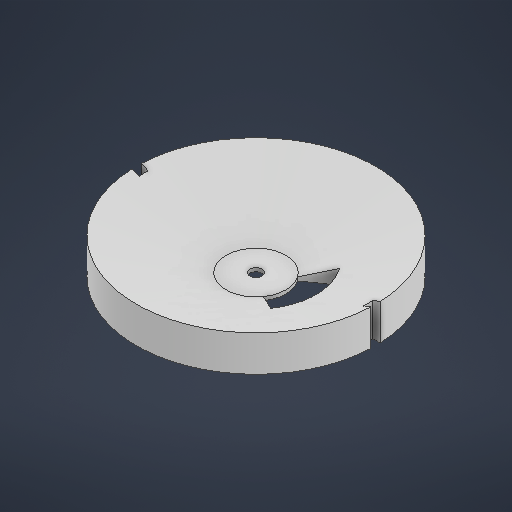
# Autodesk Inventor part: feeder
Saved by Autodesk Inventor 2025.1 (Build 291241020, 241B)
## iProperties
Created: 2024-09-17
Part Number: feeder
Material: Generic
Document SubType Name: Modeling
Designer: maxim
Density: 1 g/cm^3
Appearance: Default
Author: maxim
Autodesk Inventor part; units mm, degrees
ref_plane "YZ Plane" through (0, 0, 0) normal (1, 0, 0) x (0, 1, 0)
ref_plane "XZ Plane" through (0, 0, 0) normal (0, 1, 0) x (-1, 0, 0)
ref_plane "XY Plane" through (0, 0, 0) normal (0, 0, 1) x (1, 0, 0)
sketch "Sketch2" plane through (0, 0, 0) normal (0, 0, 1) x (1, 0, 0)
  line L0 (-50, 0) -> (-99.9, 0)
  line L1 (-99.9, 0) -> (-99.9, 30)
  line L2 (0, 0) -> (0, 50.0549)
  line L3 (-99.9, 30) -> (-25, 3)
  line L4 (-50, 0) -> (0, 0)
  line L5 (-25, 3) -> (0, 3)
  line L6 (0, 3) -> (0, 0)
  point P0 (-99.9, 15)
  dimension "d2" = 30
  dimension "d6" = 199.8
  dimension "d15" = 50
  dimension "d16" = 3
  constraints: 14 end point, 2 horizontal, 2 vertical, 1 collinear, 1 midpoint, 1 perpendicular, 1 point on line
  measures "d2" distance of L0.end L1.end
  measures "d6" diameter of point (-99.9, 15) L2
  measures "d15" diameter of L3.end L2
  measures "d16" distance of L2.start L5.end
revolve "Revolution1" add sketch "Sketch2" angle 360 about axis through (0, 0, 0) along (0, 1, 0)
sketch "Sketch3" plane through (0, 0, 0) normal (0, -1, 0) x (1, 0, 0)
  circle A0 centre (0, 0) radius 99.9 projected
  line L0 (0, 0) -> (99.8199, 4)
  line L1 (0, 0) -> (99.8199, -4)
  line L2 (0, 0) -> (99.9, 0) construction
  line L3 (11.4718, 0) -> (11.4718, -0.4597) construction
  line L4 (11.4718, 0) -> (11.4718, 0.4597) construction
  circle A1 centre (0, 0) radius 93.9
  point P0 (93.8247, 3.7598)
  point P1 (93.8247, -3.7598)
  dimension "d8" = 8
  dimension "d9" = 6
  constraints: 10 end point, 4 point on line, 3 point on circle, 1 centre point, 1 coincident, 1 collinear, 1 horizontal, 1 vertical
  measures "d8" distance of L0.end L1.end
  measures "d9" radial gap between concentric circles of A0 A1
extrude "Extrusion1" cut sketch "Sketch3" against normal through all contours A0 L1 A1 L0 picked at (97.8363, 3.4756)
pattern_circular "Circular Pattern1" count 2 over 360 about axis through (0, 16.5, 0) along (0, 1, 0) of "Extrusion1"
sketch "Sketch5" plane through (0, 3, 0) normal (0, 1, 0) x (1, 0, 0)
  point P0 (0, 0)
  point P1 (0, 0)
  constraints: 1 coincident
hole "Hole1" at (0, 3, 0) direction (0, -1, 0) diameter 10.2 end through all
sketch "Sketch6" plane through (0, 0, 0) normal (0, -1, 0) x (1, 0, 0)
  line L0 (0, 0) -> (93.9, 0) construction
  arc A0 (93.8247, -3.7598) -> (93.8247, 3.7598) centre (0, 0) ccw projected
  arc A1 (41.0395, -28.7362) -> (41.0395, 28.7362) centre (0, 0) ccw
  line L1 (0, 0) -> (41.0395, 28.7362)
  line L2 (0, 0) -> (41.0395, -28.7362)
  line L3 (16.9605, 0) -> (16.9605, 11.8759) construction
  line L4 (16.9605, 0) -> (16.9605, -11.8759) construction
  arc A2 (20.4788, -14.3394) -> (20.4788, 14.3394) centre (0, 0) ccw
  point P0 (25, 0)
  dimension "d30" = 50.1
  dimension "d31" = 70
  dimension "d32" = 25
  constraints: 10 end point, 6 point on circle, 6 point on line, 2 centre point, 2 coincident, 1 collinear, 1 horizontal, 1 perpendicular
  measures "d30" radius of A1
  measures "d31" angle of L2 L1
  measures "d32" distance of L0.start point (25, 0)
extrude "Extrusion3" cut sketch "Sketch6" against normal through all contours L2 A2 L1 A1
body "Solid1"
